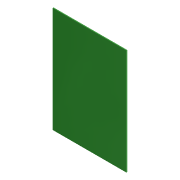
# Autodesk Inventor part: 00_PCB_Xiao_Camera_array
Saved by Autodesk Inventor 2022 (Build 260153000, 153)
## iProperties
Created: 2023-04-24
Part Number: 00_PCB_Xiao_Camera_array
Material: Generisch
Document SubType Name: Modeling
Designer: diederichbenedict
Density: 1 g/cm^3
Appearance: Glatt - Waldgrün
Author: diederichbenedict
Autodesk Inventor part; units mm, degrees
ref_plane "YZ Plane" through (0, 0, 0) normal (1, 0, 0) x (0, 1, 0)
ref_plane "XZ Plane" through (0, 0, 0) normal (0, 1, 0) x (-1, 0, 0)
ref_plane "XY Plane" through (0, 0, 0) normal (0, 0, 1) x (1, 0, 0)
sketch "Skizze1" plane through (0, 0, 0) normal (0, 0, 1) x (1, 0, 0)
  line L0 (-19.5521, 110.5093) -> (59.4809, 110.5093)
  line L1 (59.4809, 110.5093) -> (59.4809, -2.5851)
  line L2 (59.4809, -2.5851) -> (-19.5521, -2.5851)
  line L3 (-19.5521, -2.5851) -> (-19.5521, 110.5093)
  point P0 (0, 0)
  constraints: 8 end point, 2 parallel, 1 horizontal, 1 perpendicular
extrude "Extrusion1" add sketch "Skizze1" along normal blind 1
